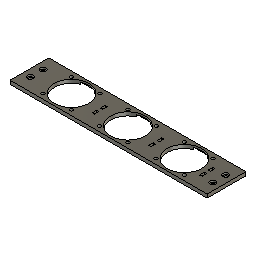
rear_fan_plate (Autodesk Fusion 360 design; units mm, degrees)
part number: 2026-08-26-09-02-38-795
Autodesk Fusion 360 part; units mm, degrees
sketch "Sketch1" plane through (0, 0, 0) normal (0, 0, 1) x (1, 0, 0)
  line L0 (-111, 0.4) -> (111, 0.4)
  line L1 (111, 0.4) -> (111, 44.05)
  line L2 (111, 44.05) -> (-111, 44.05)
  line L3 (-111, 44.05) -> (-111, 0.4)
extrude "Extrude1" add sketch "Sketch1" along normal blind 4
sketch "Sketch2" plane through (0, 0, 0) normal (0, 0, 1) x (1, 0, 0)
  circle A0 centre (-63.55, 22.225) radius 19.5
  circle A1 centre (-79.55, 6.225) radius 1.8
  circle A2 centre (-79.55, 38.225) radius 1.8
  circle A3 centre (-47.55, 6.225) radius 1.8
  circle A4 centre (-47.55, 38.225) radius 1.8
  circle A5 centre (0, 22.225) radius 19.5
  circle A6 centre (-16, 6.225) radius 1.8
  circle A7 centre (-16, 38.225) radius 1.8
  circle A8 centre (16, 6.225) radius 1.8
  circle A9 centre (16, 38.225) radius 1.8
  circle A10 centre (63.55, 22.225) radius 19.5
  circle A11 centre (47.55, 6.225) radius 1.8
  circle A12 centre (47.55, 38.225) radius 1.8
  circle A13 centre (79.55, 6.225) radius 1.8
  circle A14 centre (79.55, 38.225) radius 1.8
  circle A15 centre (-102.82, 15) radius 1.7
  circle A16 centre (-102.82, 29.45) radius 1.7
  circle A17 centre (102.82, 15) radius 1.7
  circle A18 centre (102.82, 29.45) radius 1.7
extrude "Extrude2" cut sketch "Sketch2" along normal blind 4
sketch "Sketch3" plane through (0, 0, 0) normal (0, 0, 1) x (1, 0, 0)
  line L0 (-33.03, 15) -> (-30.53, 15)
  line L1 (-30.53, 15) -> (-30.53, 20)
  line L2 (-30.53, 20) -> (-33.03, 20)
  line L3 (-33.03, 20) -> (-33.03, 15)
  line L4 (-33.03, 24.5) -> (-30.53, 24.5)
  line L5 (-30.53, 24.5) -> (-30.53, 29.5)
  line L6 (-30.53, 29.5) -> (-33.03, 29.5)
  line L7 (-33.03, 29.5) -> (-33.03, 24.5)
  line L8 (30.53, 15) -> (33.03, 15)
  line L9 (33.03, 15) -> (33.03, 20)
  line L10 (33.03, 20) -> (30.53, 20)
  line L11 (30.53, 20) -> (30.53, 15)
  line L12 (30.53, 24.5) -> (33.03, 24.5)
  line L13 (33.03, 24.5) -> (33.03, 29.5)
  line L14 (33.03, 29.5) -> (30.53, 29.5)
  line L15 (30.53, 29.5) -> (30.53, 24.5)
  line L16 (88.19, 15) -> (90.69, 15)
  line L17 (90.69, 15) -> (90.69, 20)
  line L18 (90.69, 20) -> (88.19, 20)
  line L19 (88.19, 20) -> (88.19, 15)
  line L20 (88.19, 24.5) -> (90.69, 24.5)
  line L21 (90.69, 24.5) -> (90.69, 29.5)
  line L22 (90.69, 29.5) -> (88.19, 29.5)
  line L23 (88.19, 29.5) -> (88.19, 24.5)
extrude "Extrude3" cut sketch "Sketch3" along normal blind 4
ref_plane "WorkPlane1" through (0, 0, 4) normal (0, 0, 1) x (1, 0, 0)
sketch "Sketch4" plane through (0, 0, 4) normal (0, 0, 1) x (1, 0, 0)
  circle A0 centre (-102.82, 15) radius 3.25
  circle A1 centre (-102.82, 29.45) radius 3.25
  circle A2 centre (102.82, 15) radius 3.25
  circle A3 centre (102.82, 29.45) radius 3.25
extrude "Extrude4" cut sketch "Sketch4" against normal blind 2
sketch "Sketch5" plane through (0, 0, 0) normal (0, 0, 1) x (1, 0, 0)
  line L0 (-97.6, 2) -> (97.6, 2)
  line L1 (97.6, 2) -> (97.6, 4.4)
  line L2 (97.6, 4.4) -> (-97.6, 4.4)
  line L3 (-97.6, 4.4) -> (-97.6, 2)
  line L4 (-97.6, 40.05) -> (97.6, 40.05)
  line L5 (97.6, 40.05) -> (97.6, 42.45)
  line L6 (97.6, 42.45) -> (-97.6, 42.45)
  line L7 (-97.6, 42.45) -> (-97.6, 40.05)
extrude "Extrude5" cut sketch "Sketch5" along normal blind 2
named bodies: "Rear Fan Plate"
